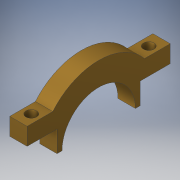
# Autodesk Inventor part: Part5
Saved by Autodesk Inventor 2019 (Build 230136000, 136)
## iProperties
Created: 2022-01-28
Part Number: Part5
Material: Generic
Document SubType Name: Modeling
Designer: Sepehr
Density: 1 g/cm^3
Appearance: Default
Author: Sepehr
Autodesk Inventor part; units mm, degrees
ref_plane "YZ Plane" through (0, 0, 0) normal (1, 0, 0) x (0, 1, 0)
ref_plane "XZ Plane" through (0, 0, 0) normal (0, 1, 0) x (-1, 0, 0)
ref_plane "XY Plane" through (0, 0, 0) normal (0, 0, 1) x (1, 0, 0)
sketch "Sketch1" plane through (0, 0, 0) normal (1, 0, 0) x (0, 1, 0)
  arc A0 (0, -1375) -> (0, 1375) centre (0, 0) ccw
  line L0 (0, -1375) -> (0, -1560)
  line L1 (0, 1375) -> (0, 1560)
  line L2 (0, 1560) -> (800, 1560)
  line L3 (800, 1560) -> (800, 2682.5)
  line L4 (0, -1560) -> (800, -1560)
  line L5 (800, -1560) -> (800, -2682.5)
  line L6 (800, -2682.5) -> (1450, -2682.5)
  line L7 (800, 2682.5) -> (1450, 2682.5)
  line L8 (1450, 2682.5) -> (1450, 1720.4651)
  line L9 (1450, -2682.5) -> (1450, -1720.4651)
  arc A1 (1450, -1720.4651) -> (1450, 1720.4651) centre (0, 0) ccw
  dimension "d3" = 185
  dimension "d4" = 185
  dimension "d5" = 800
  dimension "d6" = 1122.5
  dimension "d7" = 800
  dimension "d8" = 1122.5
  dimension "d9" = 650
  dimension "d10" = 650
  constraints: 20 end point, 4 perpendicular, 4 point on circle, 3 horizontal, 3 vertical, 2 centre point, 1 coincident
  measures "d3" distance of L0.start L0.end
  measures "d4" distance of L1.start L1.end
  measures "d5" distance of L1.end L2.end
  measures "d6" distance of L2.end L3.end
  measures "d7" distance of L0.end L4.end
  measures "d8" distance of L4.end L5.end
  measures "d9" distance of L5.end L6.end
  measures "d10" distance of L3.end L7.end
extrude "Extrusion1" add sketch "Sketch1" along normal mid plane 650
sketch "Sketch2" plane through (-325, 1450, 2682.5) normal (0, 1, 0) x (1, 0, 0)
  circle A0 centre (325, 481.0175) radius 200
  circle A1 centre (325, 4883.983) radius 200
  point P0 (325, 2682.5)
  point P1 (0, 5365)
  constraints: 2 centre point
extrude "Extrusion2" cut sketch "Sketch2" against normal blind 7000
body "Solid1"
